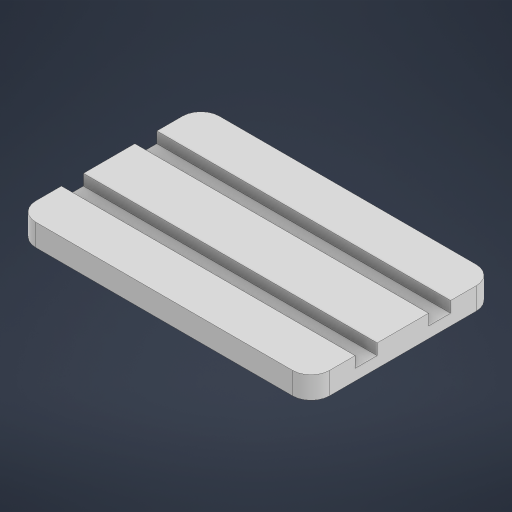
# Autodesk Inventor part: Plate
Saved by Autodesk Inventor 2023.2 (Build 272271000, 271)
## iProperties
Created: 2023-01-16
Part Number: Plate
Material: Generic
Document SubType Name: Modeling
Designer: iusti
Density: 1 g/cm^3
Appearance: Default
Author: iusti
Autodesk Inventor part; units mm, degrees
ref_plane "YZ Plane" through (0, 0, 0) normal (1, 0, 0) x (0, 1, 0)
ref_plane "XZ Plane" through (0, 0, 0) normal (0, 1, 0) x (-1, 0, 0)
ref_plane "XY Plane" through (0, 0, 0) normal (0, 0, 1) x (1, 0, 0)
sketch "Sketch2" plane through (0, 0, 0) normal (0, 1, 0) x (-1, 0, 0)
  line L0 (-40, -25) -> (40, -25)
  line L1 (40, -25) -> (40, 25)
  line L2 (40, 25) -> (-40, 25)
  line L3 (-40, 25) -> (-40, -25)
  line L4 (-40, -25) -> (40, 25) construction
  line L5 (40, -25) -> (-40, 25) construction
  line L6 (40, 13) -> (-40, 13)
  line L7 (-40, 13) -> (-40, 7)
  line L8 (-40, 7) -> (40, 7)
  line L9 (40, 7) -> (40, 13)
  line L10 (-40, -4.7355) -> (-40, -13.2457)
  line L11 (40, -14.533) -> (40, -4.7355)
  line L12 (0, 0) -> (16.546, 0)
  line L13 (40, -13) -> (-40, -13)
  line L14 (-40, -7) -> (40, -7)
  point P0 (-40, 13)
  dimension "d8" = 80
  dimension "d9" = 50
  dimension "d10" = 6
  dimension "d11" = 14
  constraints: 30 end point, 5 parallel, 4 point on line, 4 symmetric about line, 3 horizontal, 2 midpoint, 2 perpendicular
  measures "d8" distance of L2.end L1.end
  measures "d9" distance of L1.end L0.end
  measures "d10" distance between parallel lines of L6 L8
  measures "d11" distance between parallel lines of L8 L14
extrude "Extrusion1" add sketch "Sketch2" along normal blind 3
extrude "Extrusion2" add sketch "Sketch2" along normal blind 6 contours L3 L13 L1 L0 | L3 L8 L1 L14 | L3 L2 L1 L6
fillet "Fillet1" radius 5 4 edges at (-40, 3, -25) (-40, 3, 25) (40, 3, -25) (40, 3, 25)
body "Solid1"
